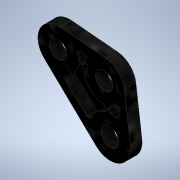
# Autodesk Inventor part: アーム 中間節 中詰め
Saved by Autodesk Inventor 2020.2 (Build 242310000, 310)
## iProperties
Created: 2020-05-09
Part Number: アーム 中間節 中詰め
Material: ABS プラスチック
Document SubType Name: Modeling
Designer: mozar
Density: 1.06 g/cm^3
Appearance: 滑らか - 黒
Mass: 2.11073 g
Surface Area: 20.5118 cm^2
Volume: 1.99125 cm^3
Author: mozar
Autodesk Inventor part; units mm, degrees
ref_plane "YZ Plane" through (0, 0, 0) normal (1, 0, 0) x (0, 1, 0)
ref_plane "XZ Plane" through (0, 0, 0) normal (0, 1, 0) x (-1, 0, 0)
ref_plane "XY Plane" through (0, 0, 0) normal (0, 0, 1) x (1, 0, 0)
sketch "スケッチ1" plane through (0, 0, 0) normal (0, 0, 1) x (1, 0, 0)
  circle A0 centre (68.955, 78.0364) radius 1.25
  arc A1 (82.2061, 79.4541) -> (58.0365, 100.3664) centre (53.5087, 70.7101) ccw
  arc A2 (58.0365, 100.3664) -> (49.826, 85.6345) centre (56.6782, 91.4695) ccw
  line L0 (78.21, 52.3031) -> (49.826, 85.6345)
  line L1 (85.7362, 40.2517) -> (78.21, 52.3031)
  arc A3 (85.7362, 40.2517) -> (86.8285, 38.9062) centre (91.6947, 43.9728) ccw
  line L2 (104.8592, 21.5887) -> (86.8285, 38.9062)
  arc A4 (104.8592, 21.5887) -> (116.6904, 27.5718) centre (109.7254, 26.6553) ccw
  line L3 (114.602, 43.4428) -> (116.6904, 27.5718)
  arc A5 (114.602, 43.4428) -> (113.6245, 46.2008) centre (107.6371, 42.5263) ccw
  line L4 (100.6394, 67.3594) -> (113.6245, 46.2008)
  arc A6 (100.6394, 67.3594) -> (89.5888, 73.7904) centre (89.1334, 60.2981) ccw
  arc A7 (82.2061, 79.4541) -> (89.5888, 73.7904) centre (89.8587, 81.7859) ccw
  circle A8 centre (89.1334, 60.2981) radius 8.525
  circle A9 centre (109.7254, 26.6553) radius 3.025
  circle A10 centre (107.6371, 42.5263) radius 3.025
  circle A11 centre (91.6947, 43.9728) radius 3.025
  circle A12 centre (56.6782, 91.4695) radius 1.25
  circle A13 centre (109.7254, 26.6553) radius 7.025
  circle A14 centre (91.6947, 43.9728) radius 7.025
  circle A15 centre (107.6371, 42.5263) radius 7.025
  line L5 (92.3295, 50.9691) -> (108.2718, 49.5226)
  point P0 (0, 0)
  point P1 (0, 0)
  constraints: 18 point on circle, 15 centre point, 12 end point, 3 coincident, 2 tangent, 48 other
extrude "押し出し1" add sketch "スケッチ1" against normal blind 4 contours A5 A15 | A14 A3 | L3 A13 L2 A14 L5 A15 | A4 A13
sketch "スケッチ2" plane through (0, 0, 0) normal (0, 0, 1) x (1, 0, 0)
  arc A0 (104.8592, 21.5887) -> (116.6904, 27.5718) centre (109.7254, 26.6553) ccw projected
  line L0 (116.6904, 27.5718) -> (114.602, 43.4428) projected
  arc A1 (114.602, 43.4428) -> (108.2718, 49.5226) centre (107.6371, 42.5263) ccw projected
  line L1 (108.2718, 49.5226) -> (92.3295, 50.9691) projected
  arc A2 (92.3295, 50.9691) -> (86.8285, 38.9062) centre (91.6947, 43.9728) ccw projected
  line L2 (86.8285, 38.9062) -> (104.8592, 21.5887) projected
  circle A3 centre (107.6371, 42.5263) radius 3.025 projected
  circle A4 centre (109.7254, 26.6553) radius 3.025 projected
  circle A5 centre (91.6947, 43.9728) radius 3.025 projected
  line L3 (108.2718, 49.5226) -> (92.3295, 50.9691) projected
  circle A6 centre (109.7254, 26.6553) radius 3.025 projected
  arc A7 (104.8592, 21.5887) -> (116.6904, 27.5718) centre (109.7254, 26.6553) ccw projected
  point P0 (0, 0)
sketch "スケッチ3" plane through (0, 0, 0) normal (0, 0, 1) x (1, 0, 0)
  arc A0 (104.8592, 21.5887) -> (116.6904, 27.5718) centre (109.7254, 26.6553) ccw projected
  line L0 (116.6904, 27.5718) -> (114.602, 43.4428) projected
  arc A1 (114.602, 43.4428) -> (108.2718, 49.5226) centre (107.6371, 42.5263) ccw projected
  line L1 (108.2718, 49.5226) -> (92.3295, 50.9691) projected
  arc A2 (92.3295, 50.9691) -> (86.8285, 38.9062) centre (91.6947, 43.9728) ccw projected
  line L2 (86.8285, 38.9062) -> (104.8592, 21.5887) projected
  circle A3 centre (107.6371, 42.5263) radius 3.025 projected
  circle A4 centre (109.7254, 26.6553) radius 3.025 projected
  circle A5 centre (91.6947, 43.9728) radius 3.025 projected
  arc A6 (106.9373, 23.7524) -> (113.716, 27.1804) centre (109.7254, 26.6553) ccw
  line L3 (113.716, 27.1804) -> (111.6277, 43.0514)
  arc A7 (111.6277, 43.0514) -> (108.0008, 46.5349) centre (107.6371, 42.5263) ccw
  line L4 (108.0008, 46.5349) -> (92.0584, 47.9813)
  arc A8 (92.0584, 47.9813) -> (88.9066, 41.0699) centre (91.6947, 43.9728) ccw
  line L5 (88.9066, 41.0699) -> (106.9373, 23.7524)
  line L6 (104.8592, 21.5887) -> (86.8285, 38.9062) projected
  circle A9 centre (91.6947, 43.9728) radius 7.025
  line L7 (114.602, 43.4428) -> (116.6904, 27.5718) projected
  circle A10 centre (107.6371, 42.5263) radius 7.025
  circle A11 centre (109.7254, 26.6553) radius 7.025
  point P0 (0, 0)
  point P1 (102.7848, 27.7407)
  point P2 (112.9649, 32.8888)
  point P3 (112.3788, 37.343)
  point P4 (102.2667, 47.0551)
  point P5 (97.7925, 47.4611)
  point P6 (93.0592, 37.0816)
  dimension "d2" = 3
  constraints: 6 end point, 6 point on circle, 3 centre point, 3 coincident, 14 other
  measures "d2" distance between parallel lines of L2 L5
extrude "押し出し2" cut sketch "スケッチ3" against normal blind 3.5 contours L5 A9 L4 A10 L3 A11
sketch "スケッチ4" plane through (0, 0, 0) normal (0, 0, 1) x (1, 0, 0)
  line L0 (112.3788, 37.343) -> (112.9649, 32.8888) projected
  arc A0 (112.9649, 32.8888) -> (102.7848, 27.7407) centre (109.7254, 26.6553) ccw projected
  line L1 (102.7848, 27.7407) -> (93.0592, 37.0816) projected
  arc A1 (93.0592, 37.0816) -> (97.7925, 47.4611) centre (91.6947, 43.9728) ccw projected
  line L2 (97.7925, 47.4611) -> (102.2667, 47.0551) projected
  arc A2 (102.2667, 47.0551) -> (112.3788, 37.343) centre (107.6371, 42.5263) ccw projected
  arc A3 (104.8592, 21.5887) -> (116.6904, 27.5718) centre (109.7254, 26.6553) ccw projected
  line L3 (116.6904, 27.5718) -> (114.602, 43.4428) projected
  arc A4 (114.602, 43.4428) -> (108.2718, 49.5226) centre (107.6371, 42.5263) ccw projected
  line L4 (108.2718, 49.5226) -> (92.3295, 50.9691) projected
  arc A5 (92.3295, 50.9691) -> (86.8285, 38.9062) centre (91.6947, 43.9728) ccw projected
  line L5 (86.8285, 38.9062) -> (104.8592, 21.5887) projected
  circle A6 centre (107.6371, 42.5263) radius 3.025 projected
  circle A7 centre (109.7254, 26.6553) radius 3.025 projected
  circle A8 centre (91.6947, 43.9728) radius 3.025 projected
  arc A9 (102.2667, 47.0551) -> (112.3788, 37.343) centre (107.6371, 42.5263) ccw projected
  line L6 (91.6947, 43.9728) -> (107.6371, 42.5263) construction
  line L7 (91.6722, 43.7238) -> (107.6145, 42.2774)
  line L8 (107.6597, 42.7753) -> (91.7173, 44.2218)
  arc A10 (91.7173, 44.2218) -> (91.6722, 43.7238) centre (91.6947, 43.9728) ccw
  arc A11 (107.6145, 42.2774) -> (107.6597, 42.7753) centre (107.6371, 42.5263) ccw
  line L9 (107.6371, 42.5263) -> (109.7254, 26.6553) construction
  line L10 (107.3892, 42.4937) -> (109.4776, 26.6227)
  line L11 (109.9733, 26.688) -> (107.8849, 42.559)
  arc A12 (107.8849, 42.559) -> (107.3892, 42.4937) centre (107.6371, 42.5263) ccw
  arc A13 (109.4776, 26.6227) -> (109.9733, 26.688) centre (109.7254, 26.6553) ccw
  point P0 (0, 0)
  point P1 (99.6659, 43.2496)
  point P2 (108.6812, 34.5908)
  point P3 (109.0574, 33.6485)
  point P4 (108.8008, 35.5984)
  point P5 (108.3051, 35.5332)
  point P6 (108.5617, 33.5833)
  point P7 (100.6678, 43.4097)
  point P8 (98.7092, 43.5874)
  point P9 (98.664, 43.0895)
  point P10 (100.6227, 42.9117)
  dimension "d9" = 0.5
  dimension "d10" = 0.5
  constraints: 16 end point, 8 point on circle, 8 tangent, 4 centre point, 2 midpoint, 2 parallel
  measures "d9" diameter of A11
  measures "d10" diameter of A13
extrude "押し出し3" add sketch "スケッチ4" against normal blind 4 contours L11 A0 L10 A2 | L7 A1 L8 A2
fillet "フィレット1" radius 1 14 edges at (97.7925, 47.4611, -1.75) (102.2667, 47.0551, -1.75) (98.7092, 43.5874, -1.75) (98.664, 43.0895, -1.75) (100.6678, 43.4097, -1.75) (100.6227, 42.9117, -1.75) (93.0592, 37.0816, -1.75) (112.3788, 37.343, -1.75) (112.9649, 32.8888, -1.75) (108.8008, 35.5984, -1.75) (108.3051, 35.5332, -1.75) (109.0574, 33.6485, -1.75) (108.5617, 33.5833, -1.75) (102.7848, 27.7407, -1.75)
